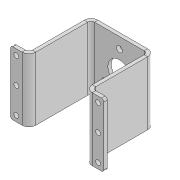
# Autodesk Inventor part: CCM_Motor_Mount_A
Saved by Autodesk Inventor 2020 (Build 240168000, 168)
## iProperties
Created: 2021-12-08
Part Number: CCM_Motor_Mount_A
Material: 一般
Document SubType Name: Sheet Metal
Designer: magnarecta
Density: 1 g/cm^3
Sheet Metal Rule: Default_mm
Appearance: 既定
Author: magnarecta
Autodesk Inventor part; units mm, degrees
ref_plane "YZ Plane" through (0, 0, 0) normal (1, 0, 0) x (0, 1, 0)
ref_plane "XZ Plane" through (0, 0, 0) normal (0, 1, 0) x (-1, 0, 0)
ref_plane "XY Plane" through (0, 0, 0) normal (0, 0, 1) x (1, 0, 0)
sketch "スケッチ1" plane through (0, 0, 0) normal (0, 0, 1) x (1, 0, 0)
  line L0 (27.5, -27.5) -> (-27.5, -27.5)
  line L1 (-27.5, -27.5) -> (-27.5, 27.5)
  line L2 (-27.5, 27.5) -> (27.5, 27.5)
  line L3 (27.5, 27.5) -> (27.5, -27.5)
  line L4 (27.5, -27.5) -> (-27.5, 27.5) construction
  line L5 (-27.5, -27.5) -> (27.5, 27.5) construction
  point P0 (0, 0)
  dimension "d0" = 55
  dimension "d1" = 55
  measures "d0" distance of L1.end L2.end
  measures "d1" distance of L0.end L1.end
extrude "プレート1" add sketch "スケッチ1" along normal blind 3
sketch "スケッチ2" plane through (0, 0, 3) normal (0, 0, 1) x (1, 0, 0)
  line L0 (-27.5, -27.5) -> (-27.5, 27.5) projected
  line L1 (27.5, -27.5) -> (-27.5, -27.5) projected
  line L2 (27.5, 27.5) -> (27.5, -27.5) projected
  line L3 (-27.5, 27.5) -> (27.5, 27.5) projected
  circle A0 centre (0, 0) radius 18
  point P0 (0, 18)
  point P1 (-18, 0)
  point P2 (0, -18)
  point P3 (18, 0)
  point P4 (-12.728, -12.7278)
  point P5 (12.728, -12.7278)
  dimension "d3" = 36
  dimension "d54" = 25.456
  constraints: 3 point on circle, 1 centre point, 1 coincident, 1 horizontal alignment, 1 vertical alignment
  measures "d3" diameter of A0
  measures "d54" distance of point (12.728, -12.728) A0.end
hole "穴1" at (0, 18, 3) at (12.728, -12.7278, 3) at (-12.728, -12.7278, 3) direction (0, 0, -1) diameter 5.2 end through all
sketch "スケッチ3" plane through (0, 0, 3) normal (0, 0, 1) x (1, 0, 0)
  circle A0 centre (0, 0) radius 10
  dimension "d15" = 20
  constraints: 1 centre point, 1 coincident
  measures "d15" diameter of A0
extrude "押し出し1" cut sketch "スケッチ3" against normal blind 10
sketch "スケッチ4" plane through (-24.5, -27.5, 0) normal (-1, 0, 0) x (0, -1, 0)
  line L0 (-55, 0) -> (0, 0)
  line L1 (0, 0) -> (0, 57)
  line L2 (0, 57) -> (-55, 57)
  line L3 (-55, 57) -> (-55, 0)
  constraints: 6 end point, 1 horizontal, 1 perpendicular, 1 vertical
edge flange "フランジ1" height 57 angle 90 thickness 3 bend radius 3 thickness toward (-1, 0, 0) relief tear relief width 3 relief depth 1.5 corner gap 3 corner form 0 edges at (-27.5, 0, 3) (27.5, 0, 3) wall of the first edge with corners at (-24.5, 27.5, 0) (-24.5, -27.5, 0) (-24.5, -27.5, 57) (-24.5, 27.5, 57)
bend "曲げ1"
corner "コーナー1"
sketch "スケッチ5" plane through (24.5, -27.5, 54) normal (0, 0, 1) x (1, 0, 0)
  line L0 (0, 55) -> (0, 0)
  line L1 (0, 0) -> (16, 0)
  line L2 (16, 0) -> (16, 55)
  line L3 (16, 55) -> (0, 55)
  constraints: 6 end point, 1 horizontal, 1 perpendicular, 1 vertical
edge flange "フランジ2" height 16 angle 90 thickness 3 bend radius 3 thickness toward (0, 0, 1) relief tear relief width 3 relief depth 1.5 corner gap 3 corner form 0 edges at (27.5, 0, 57) (-27.5, 0, 57) wall of the first edge with corners at (24.5, 27.5, 54) (24.5, -27.5, 54) (40.5, -27.5, 54) (40.5, 27.5, 54)
bend "曲げ2"
corner "コーナー2"
fillet "フィレット1" radius 2 4 edges at (40.5, 27.5, 55.5) (40.5, -27.5, 55.5) (-40.5, -27.5, 55.5) (-40.5, 27.5, 55.5)
sketch "スケッチ8" plane through (-30.5, -27.5, 57) normal (0, 0, 1) x (1, 0, 0)
  arc A0 (-8, 55) -> (-10, 53) centre (-8, 53) ccw projected
  line L0 (-10, 2) -> (-10, 53) projected
  arc A1 (-10, 2) -> (-8, 0) centre (-8, 2) ccw projected
  line L1 (0, 0) -> (-8, 0) projected
  line L2 (0, 0) -> (0, 55) projected
  line L3 (-8, 55) -> (0, 55) projected
  arc A2 (69, 0) -> (71, 2) centre (69, 2) ccw projected
  line L4 (71, 53) -> (71, 2) projected
  arc A3 (71, 53) -> (69, 55) centre (69, 53) ccw projected
  line L5 (61, 55) -> (69, 55) projected
  line L6 (61, 55) -> (61, 0) projected
  line L7 (69, 0) -> (61, 0) projected
  line L8 (-5, 50) -> (66, 50)
  line L9 (66, 50) -> (66, 5)
  line L10 (66, 5) -> (-5, 5)
  line L11 (-5, 5) -> (-5, 50)
  point P0 (30.5, 27.5)
  point P1 (-5, 27.5)
  point P2 (66, 27.5)
  dimension "d55" = 5
  dimension "d56" = 5
  dimension "d57" = 5
  dimension "d58" = 5
  constraints: 8 end point, 2 midpoint, 2 parallel, 1 horizontal, 1 perpendicular
  measures "d55" distance between parallel lines of L11 L0
  measures "d56" distance between parallel lines of L5 L8
  measures "d57" distance between parallel lines of L10 L7
  measures "d58" distance between parallel lines of L4 L9
hole "穴3" at (-35.5, 0, 57) at (35.5, 0, 57) at (-35.5, -22.5, 57) at (-35.5, 22.5, 57) at (35.5, -22.5, 57) at (35.5, 22.5, 57) direction (0, 0, -1) diameter 4.2 end through all
equation "\"d13\" = Thickness"
equation "\"d64\" = Thickness"
equation "\"d2\" = Thickness"
equation "\"d18\" = BendReliefWidth"
equation "\"d19\" = BendReliefDepth"
equation "\"d20\" = MinimumRemnant"
equation "\"d21\" = TransitionRadius"
equation "\"d24\" = BendRadius"
equation "\"d25\" = CornerReliefSize"
equation "\"d26\" = GapSize"
equation "\"d27\" = JacobiRadiusSize"
equation "\"d28\" = BendReliefWidth"
equation "\"d29\" = BendReliefDepth"
equation "\"d30\" = MinimumRemnant"
equation "\"d31\" = TransitionRadius"
equation "\"d34\" = BendRadius"
equation "\"d35\" = CornerReliefSize"
equation "\"d36\" = GapSize"
equation "\"d37\" = JacobiRadiusSize"
equation "\"BendRadius\" = Thickness"
equation "\"BendReliefWidth\" = Thickness"
equation "\"BendReliefDepth\" = 0.5 * Thickness"
equation "\"CornerReliefSize\" = 4 * Thickness"
equation "\"MinimumRemnant\" = 2 * Thickness"
equation "\"TransitionRadius\" = BendRadius"
equation "\"JacobiRadiusSize\" = BendRadius"
equation "\"GapSize\" = Thickness"
equation "\"Thickness\" = 3"
